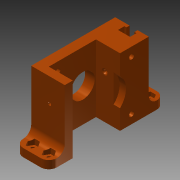
# Autodesk Inventor part: filament drive mount
Saved by Autodesk Inventor 2013 (Build 170138000, 138)
## iProperties
Created: 2013-08-05
Part Number: filament drive mount
Material: Generic
Document SubType Name: Modeling
Designer: employee
Density: 1 g/cm^3
Mass: 27.1634 g
Surface Area: 106.905 cm^2
Volume: 27.1634 cm^3
Author: employee
Autodesk Inventor part; units mm, degrees
ref_plane "YZ Plane" through (0, 0, 0) normal (1, 0, 0) x (0, 1, 0)
ref_plane "XZ Plane" through (0, 0, 0) normal (0, 1, 0) x (-1, 0, 0)
ref_plane "XY Plane" through (0, 0, 0) normal (0, 0, 1) x (1, 0, 0)
sketch "Sketch1" plane through (0, 0, 0) normal (0, 0, 1) x (1, 0, 0)
  line L0 (0, -21.25) -> (0, 21.25)
  line L1 (0, 21.25) -> (20, 21.25)
  line L2 (20, 21.25) -> (20, 8.25)
  line L3 (20, 8.25) -> (5, 8.25)
  line L4 (5, 8.25) -> (5, -21.25)
  line L5 (5, -21.25) -> (0, -21.25)
  line L6 (0, 21.25) -> (20, 21.25)
  line L7 (20, 21.25) -> (20, 26.25)
  line L8 (20, 26.25) -> (0, 26.25)
  line L9 (0, 26.25) -> (0, 21.25)
  line L10 (0, -21.25) -> (20, -21.25)
  line L11 (20, -21.25) -> (20, -26.25)
  line L12 (20, -26.25) -> (0, -26.25)
  line L13 (0, -26.25) -> (0, -21.25)
  point P0 (0, 0)
  point P1 (0, 0)
  dimension "d0" = 5
  dimension "d2" = 42.5
  dimension "d3" = 29.5
  dimension "d4" = 15
  constraints: 28 end point, 8 parallel, 3 perpendicular, 2 equal length, 2 horizontal, 2 vertical alignment, 1 coincident, 1 midpoint, 1 vertical
  measures "d0" distance of L4.end L0.start
  measures "d2" distance of L0.start L0.end
  measures "d3" distance of L3.end L4.end
  measures "d4" distance of L2.end L3.end
extrude "Extrusion1" add sketch "Sketch1" along normal blind 42
sketch "Sketch2" plane through (0, 26.25, 0) normal (0, 1, 0) x (1, 0, 0)
  line L0 (20, 0) -> (20, -42) projected
  line L1 (0, 0) -> (20, 0)
  line L2 (20, 0) -> (20, -5)
  line L3 (20, -5) -> (0, -5)
  line L4 (0, -5) -> (0, 0)
  dimension "d7" = 5
  constraints: 8 end point, 2 parallel, 1 horizontal, 1 perpendicular, 1 point on line
  measures "d7" distance of L1.end L2.end
extrude "Extrusion2" add sketch "Sketch2" along normal blind 10
sketch "Sketch3" plane through (0, -26.25, 0) normal (0, -1, 0) x (1, 0, 0)
  line L0 (0, 0) -> (0, 42) projected
  line L1 (20, 0) -> (0, 0)
  line L2 (0, 0) -> (0, 5)
  line L3 (0, 5) -> (20, 5)
  line L4 (20, 5) -> (20, 0)
  dimension "d11" = 5
  constraints: 8 end point, 2 parallel, 1 horizontal, 1 perpendicular, 1 point on line
  measures "d11" distance of L1.end L2.end
extrude "Extrusion3" add sketch "Sketch3" along normal blind 10
sketch "Sketch4" plane through (0, -26.25, 5) normal (0, 0, 1) x (1, 0, 0)
  line L0 (0, 0) -> (0, -10) projected
  line L1 (20, -10) -> (0, -10) projected
  line L2 (20, 0) -> (20, -10) projected
  line L3 (5, -5) -> (15, -5)
  line L4 (20, 52.5) -> (0, 52.5) projected
  line L5 (20, 52.5) -> (20, 62.5) projected
  line L6 (0, 62.5) -> (20, 62.5) projected
  line L7 (0, 52.5) -> (0, 62.5) projected
  line L8 (5, 57.5) -> (15, 57.5)
  circle A0 centre (15, -5) radius 1.55
  circle A1 centre (5, -5) radius 1.55
  circle A2 centre (5, 57.5) radius 1.55
  circle A3 centre (15, 57.5) radius 1.55
  point P0 (0, 26.25)
  point P1 (10, -5)
  point P2 (10, -10)
  point P3 (20, -5)
  point P4 (10, 57.5)
  point P5 (20, 57.5)
  point P6 (10, 62.5)
  dimension "d15" = 5
  dimension "d16" = 3.1
  constraints: 6 midpoint, 4 centre point, 4 coincident, 4 end point, 3 equal radius, 2 horizontal alignment, 2 vertical alignment, 1 horizontal, 1 parallel, 1 perpendicular
  measures "d15" distance from line of L0 L3.start
  measures "d16" diameter of A0
extrude "Extrusion4" cut sketch "Sketch4" against normal through all contours A0 | A1 | A2 | A3
sketch "Sketch5" plane through (0, 26.25, 5) normal (0, 0, 1) x (1, 0, 0)
  circle A0 centre (5, 5) radius 1.55 projected
  circle A1 centre (15, 5) radius 1.55 projected
  line L0 (8.2332, 5) -> (6.6166, 2.2)
  line L1 (6.6166, 2.2) -> (3.3834, 2.2)
  line L2 (3.3834, 2.2) -> (1.7668, 5)
  line L3 (1.7668, 5) -> (3.3834, 7.8)
  line L4 (3.3834, 7.8) -> (6.6166, 7.8)
  line L5 (6.6166, 7.8) -> (8.2332, 5)
  line L6 (11.7668, 5) -> (13.3834, 7.8)
  line L7 (13.3834, 7.8) -> (16.6166, 7.8)
  line L8 (16.6166, 7.8) -> (18.2332, 5)
  line L9 (18.2332, 5) -> (16.6166, 2.2)
  line L10 (16.6166, 2.2) -> (13.3834, 2.2)
  line L11 (13.3834, 2.2) -> (11.7668, 5)
  circle A2 centre (15, -57.5) radius 1.55 projected
  circle A3 centre (5, -57.5) radius 1.55 projected
  line L12 (0, -52.5) -> (20, -52.5) projected
  line L13 (0, -52.5) -> (0, -62.5) projected
  line L14 (20, -62.5) -> (0, -62.5) projected
  line L15 (20, -52.5) -> (20, -62.5) projected
  line L16 (8.2332, -57.5) -> (6.6166, -60.3)
  line L17 (6.6166, -60.3) -> (3.3834, -60.3)
  line L18 (3.3834, -60.3) -> (1.7668, -57.5)
  line L19 (1.7668, -57.5) -> (3.3834, -54.7)
  line L20 (3.3834, -54.7) -> (6.6166, -54.7)
  line L21 (6.6166, -54.7) -> (8.2332, -57.5)
  line L22 (11.7668, -57.5) -> (13.3834, -54.7)
  line L23 (13.3834, -54.7) -> (16.6166, -54.7)
  line L24 (16.6166, -54.7) -> (18.2332, -57.5)
  line L25 (18.2332, -57.5) -> (16.6166, -60.3)
  line L26 (16.6166, -60.3) -> (13.3834, -60.3)
  line L27 (13.3834, -60.3) -> (11.7668, -57.5)
  point P0 (0, -26.25)
  point P1 (15, -54.7)
  dimension "d19" = 5.6
  constraints: 48 end point, 4 coincident, 3 equal length, 3 horizontal, 1 horizontal alignment, 1 midpoint, 52 other
  measures "d19" distance between parallel lines of L17 L20
extrude "Extrusion5" cut sketch "Sketch5" against normal blind 2.5 contours L0 L1 L2 L3 L4 L5 | L6 L7 L8 L9 L10 L11 | L16 L17 L18 L19 L20 L21 | L22 L23 L24 L25 L26 L27
sketch "Sketch6" plane through (0, -26.25, 42) normal (-1, 0, 0) x (0, 0, 1)
  line L0 (0, 52.5) -> (0, 0) projected
  line L1 (-42, 26.25) -> (0, 26.25)
  line L2 (-36.5, 41.75) -> (-5.5, 41.75)
  line L3 (-5.5, 41.75) -> (-5.5, 10.75)
  line L4 (-5.5, 10.75) -> (-36.5, 10.75)
  line L5 (-36.5, 10.75) -> (-36.5, 41.75)
  circle A0 centre (-36.5, 41.75) radius 1.55
  circle A1 centre (-5.5, 41.75) radius 1.55
  circle A2 centre (-36.5, 10.75) radius 1.55
  circle A3 centre (-5.5, 10.75) radius 1.55
  point P0 (-21, 26.25)
  dimension "d23" = 31
  dimension "d24" = 3.1
  constraints: 10 end point, 4 centre point, 4 coincident, 3 equal radius, 2 midpoint, 1 horizontal, 9 other
  measures "d23" distance of L2.end L3.end
  measures "d24" diameter of A3
extrude "Extrusion6" cut sketch "Sketch6" against normal through all contours A2 L4 L5 | L5 L4 A2 | A0 L2 L5 | L5 L2 A0 | A1 L2 L3 | L3 L2 A1 | A3 L4 L3 | L3 L4 A3
sketch "Sketch8" plane through (5, -21.25, 0) normal (0, 1, 0) x (1, 0, 0)
  line L0 (15, 0) -> (15, -42) projected
  line L1 (15, 0) -> (0, 0) projected
  circle A0 centre (5.5, -27.135) radius 1 projected
  circle A1 centre (5.5, -14.885) radius 1 projected
  line L2 (0, -37.01) -> (15, -37.01) projected
  line L3 (0, -5.01) -> (0, -37.01) projected
  line L4 (15, -5.01) -> (0, -5.01) projected
  line L5 (15, -37.01) -> (15, -5.01) projected
  circle A2 centre (5.5, -27.135) radius 1
  point P0 (-5, 0)
  point P1 (15, -21)
  point P2 (7.5, 0)
  dimension "d62" = 2
  constraints: 2 midpoint, 1 centre point, 1 coincident
  measures "d62" diameter of A2
extrude "Extrusion8" cut sketch "Sketch8" along normal through all both and the other way through all contours A0
sketch "Sketch10" plane through (0, -26.25, 42) normal (-1, 0, 0) x (0, 0, 1)
  circle A0 centre (-36.5, 41.75) radius 3.25 projected
  circle A1 centre (-5.5, 10.75) radius 1.55 projected
  line L0 (-36.5, 41.75) -> (-5.5, 10.75)
  circle A2 centre (-21, 26.25) radius 7.5
  point P0 (-42, 26.25)
  dimension "d38" = 15
  constraints: 2 end point, 1 centre point, 1 midpoint
  measures "d38" diameter of A2
extrude "Extrusion9" cut sketch "Sketch10" against normal through all contours A2 L0 | L0 A2
sketch "Sketch15" plane through (0, -26.25, 42) normal (-1, 0, 0) x (0, 0, 1)
  circle A0 centre (-21, 26.25) radius 7.5 projected
  circle A1 centre (-5.5, 41.75) radius 1.55 projected
  circle A2 centre (-5.5, 10.75) radius 1.55 projected
  circle A3 centre (-36.5, 10.75) radius 1.55 projected
  circle A4 centre (-36.5, 41.75) radius 1.55 projected
  line L0 (-42, -10) -> (-42, 62.5) projected
  line L1 (-37, -10) -> (-42, -10) projected
  line L2 (-37, 0) -> (-37, -10) projected
  line L3 (-37, 0) -> (0, 0) projected
  line L4 (0, 52.5) -> (0, 0) projected
  line L5 (-37, 52.5) -> (0, 52.5) projected
  line L6 (-37, 52.5) -> (-37, 62.5) projected
  line L7 (-42, 62.5) -> (-37, 62.5) projected
  point P0 (-42, 26.25)
extrude "Extrusion14" add sketch "Sketch15" along normal blind 1
fillet "Fillet3" radius 5 2 edges at (9.5, -26.25, 5) (9.5, 26.25, 5)
sketch "Sketch17" plane through (20, 8.25, 42) normal (1, 0, 0) x (0, 0, -1)
  arc A0 (37, -39.5) -> (32, -34.5) centre (32, -39.5) ccw projected
  line L0 (32, -34.5) -> (0, -34.5) projected
  line L1 (0, -34.5) -> (0, -29.5) projected
  line L2 (0, -29.5) -> (42, -29.5) projected
  line L3 (42, -29.5) -> (42, -44.5) projected
  circle A1 centre (5.5, 7.25) radius 1.55 projected
  line L4 (42, 28) -> (42, 0) projected
  line L5 (42, 0) -> (0, 0) projected
  line L6 (0, 0) -> (0, 18) projected
  line L7 (0, 18) -> (32, 18) projected
  circle A2 centre (36.5, 7.25) radius 1.55 projected
  circle A3 centre (21, -8.25) radius 7.5 projected
  circle A4 centre (21, -8.25) radius 12
  arc A5 (32, 18) -> (37, 23) centre (32, 23) ccw projected
  line L8 (37, 23) -> (37, 28) projected
  line L9 (37, 28) -> (42, 28) projected
  line L10 (42, -44.5) -> (37, -44.5) projected
  line L11 (37, -44.5) -> (37, -39.5) projected
  point P0 (42, -8.25)
  dimension "d74" = 24
  constraints: 1 centre point, 1 coincident
  measures "d74" diameter of A4
extrude "Extrusion16" cut sketch "Sketch17" against normal blind 4 contours A4 L5 | L5 A4 | A3
fillet "Fillet4" radius 5 4 edges at (-1, 36.25, 2.5) (20, 36.25, 2.5) (-1, -36.25, 2.5) (20, -36.25, 2.5)
sketch "Sketch18" plane through (-1, 26.25, 42) normal (0, 1, 0) x (1, 0, 0)
  line L0 (21, 0) -> (0, 0)
  line L1 (15.25, 12.6999) -> (11.5, 10.5349)
  line L2 (11.5, 10.5349) -> (7.75, 12.6999)
  line L3 (7.75, 12.6999) -> (7.75, 17.0301)
  line L4 (7.75, 17.0301) -> (11.5, 19.1951)
  line L5 (11.5, 19.1951) -> (15.25, 17.0301)
  line L6 (15.25, 17.0301) -> (15.25, 12.6999)
  line L7 (7.75, 12.6999) -> (7.75, 0)
  line L8 (15.25, 12.6999) -> (15.25, 0)
  point P0 (1, 42)
  point P1 (11.5, 14.865)
  dimension "d79" = 7.5
  constraints: 18 end point, 2 perpendicular, 2 point on line, 1 vertical, 13 other
  measures "d79" distance between parallel lines of L5 L2
extrude "Extrusion17" cut sketch "Sketch18" against normal blind 6
sketch "Sketch19" plane through (-1, 26.25, 10) normal (0, 1, 0) x (1, 0, 0)
  line L0 (7.75, -32) -> (7.75, -14.9699) projected
  line L1 (7.75, -14.9699) -> (11.5, -12.8049) projected
  line L2 (11.5, -12.8049) -> (15.25, -14.9699) projected
  line L3 (15.25, -14.9699) -> (15.25, -32) projected
  line L4 (21, -32) -> (15.25, -32) projected
  line L5 (21, 0) -> (21, -32) projected
  line L6 (0, 0) -> (21, 0) projected
  line L7 (0, -32) -> (0, 0) projected
  line L8 (7.75, -32) -> (0, -32) projected
  circle A0 centre (11.5, -17.135) radius 1 projected
  circle A1 centre (11.5, -17.135) radius 2.5
  line L9 (7.75, -32) -> (15.7931, -32)
  point P0 (1, 10)
  dimension "d83" = 5
  constraints: 2 end point, 1 centre point, 1 coincident, 1 point on line
  measures "d83" diameter of A1
extrude "Extrusion18" add sketch "Sketch19" against normal blind 2 contours L0 L1 L2 L3 L9
fillet "Fillet5" radius 1 1 edges at (9.5, 8.25, 27.135)
sketch "Sketch20" plane through (-1, 26.25, 42) normal (0, 1, 0) x (1, 0, 0)
  circle A0 centre (11.5, 14.865) radius 2.5 projected
  line L0 (21, 0) -> (0, 0) projected
  line L1 (9, 14.865) -> (9, 0)
  line L2 (14, 14.865) -> (14, 0)
  point P0 (1, 42)
  constraints: 4 end point, 2 perpendicular, 2 point on circle, 2 point on line, 2 tangent
extrude "Extrusion19" cut sketch "Sketch20" against normal up to surface (6 mm away) contours L2 L0 L1 A0
body "Solid1"
